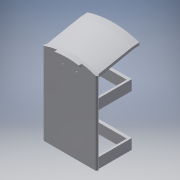
# Autodesk Inventor part: baseBateria
Saved by Autodesk Inventor 2017 (Build 210142000, 142)
## iProperties
Part Number: baseBateria
Material: Genérico
Document SubType Name: Modeling
Designer: Roberto
Density: 1 g/cm^3
Appearance: Valor por defecto
Author: Roberto
Autodesk Inventor part; units mm, degrees
ref_plane "XZ Plane" through (0, 0, 0) normal (0, 1, 0) x (-1, 0, 0)
ref_plane "XY Plane" through (0, 0, 0) normal (0, 0, 1) x (1, 0, 0)
sketch "Boceto1" plane through (0, 0, 0) normal (0, 1, 0) x (-1, 0, 0)
  line L0 (4.95, 0) -> (4.95, 8.1056)
  line L1 (-0.15, 0) -> (-0.15, 8.1056)
  arc A0 (4.95, 8.0532) -> (-0.15, 8.0532) centre (2.4, 1) ccw
  line L2 (-0.15, 0) -> (4.8, 0)
  line L3 (4.95, 0) -> (4.5, 0)
  line L4 (4.65, 0) -> (4.65, 1)
  line L5 (4.65, 1) -> (4.95, 1)
  line L6 (4.95, 5) -> (4.65, 5)
  line L7 (4.65, 5) -> (4.65, 6)
  line L8 (4.65, 6) -> (4.95, 6)
  line L9 (0.15, 0) -> (0.15, 1)
  line L10 (0.15, 1) -> (-0.15, 1)
  line L11 (-0.15, 5) -> (0.15, 5)
  line L12 (0.15, 5) -> (0.15, 6)
  line L13 (0.15, 6) -> (-0.15, 6)
  line L14 (0, 0) -> (1.4, 0)
  circle A1 centre (3.075, 7.5) radius 0.15
  circle A2 centre (1.725, 7.5) radius 0.15
  line L15 (2.55, 8.1985) -> (2.55, 0)
  line L16 (2.25, 8.1985) -> (2.25, 0)
  line L17 (0.9, 8.0485) -> (0.9, 0)
  line L18 (1.2, 8.1034) -> (1.2, 0)
  line L19 (3.9, 8.0485) -> (3.9, 0)
  line L20 (3.6, 8.1034) -> (3.6, 0)
  arc A3 (4.95, 7.7532) -> (-0.15, 7.7532) centre (2.4, 0.7) ccw
  line L21 (4.8, 0) -> (4.95, 0)
  line L22 (4.95, 8.0532) -> (4.95, 0)
  line L23 (4.95, 0) -> (-0.15, 0)
  constraints: 46 end point, 12 point on line, 10 point on circle, 4 centre point, 1 horizontal, 1 perpendicular, 1 vertical, 10 other
extrude "Extrusión1" add sketch "Boceto1" along normal blind 0.3
sketch "Boceto2" plane through (0, 0.3, 0) normal (0, 1, 0) x (1, 0, 0)
  line L0 (-4.8, 0) -> (-4.8, -8.1056)
  line L1 (0, 0) -> (0, -8.1056)
  arc A0 (-4.8, -8.1056) -> (0, -8.1056) centre (-2.4, -1) ccw
  line L2 (0, 0) -> (-4.8, 0)
  line L3 (-4.8, 0) -> (-4.5, 0)
  line L4 (-4.5, 0) -> (-4.5, -1)
  line L5 (-4.5, -1) -> (-4.8, -1)
  line L6 (-4.8, -5) -> (-4.5, -5)
  line L7 (-4.5, -5) -> (-4.5, -6)
  line L8 (-4.5, -6) -> (-4.8, -6)
  line L9 (-0.3, 0) -> (-0.3, -1)
  line L10 (-0.3, -1) -> (0, -1)
  line L11 (0, -5) -> (-0.3, -5)
  line L12 (-0.3, -5) -> (-0.3, -6)
  line L13 (-0.3, -6) -> (0, -6)
  line L14 (0, 0) -> (-1.4, 0)
  circle A1 centre (-3.075, -7.5) radius 0.15
  circle A2 centre (-1.725, -7.5) radius 0.15
  line L15 (-2.55, -7.8056) -> (-2.55, 0)
  line L16 (-2.25, -7.8056) -> (-2.25, 0)
  line L17 (-0.9, -7.8056) -> (-0.9, 0)
  line L18 (-1.2, -7.8056) -> (-1.2, 0)
  line L19 (-3.9, -7.8056) -> (-3.9, 0)
  line L20 (-3.6, -7.8056) -> (-3.6, 0)
  arc A3 (-4.8, -7.8056) -> (0, -7.8056) centre (-2.4, -0.7) ccw
  line L21 (-3.6, -7.8056) -> (-3.9, -7.8056)
  line L22 (-0.9, -7.8056) -> (-1.2, -7.8056)
  line L23 (-2.25, -7.8056) -> (-2.55, -7.8056)
  point P0 (0, 0)
  point P1 (-2.55, -8.1985)
  point P2 (-2.25, -8.1985)
  point P3 (-0.9, -8.0485)
  point P4 (-1.2, -8.1034)
  point P5 (-3.9, -8.0485)
  point P6 (-3.6, -8.1034)
  constraints: 46 end point, 11 point on line, 10 point on circle, 4 centre point, 3 horizontal, 12 other
extrude "Extrusión2" add sketch "Boceto2" along normal blind 0.3 contours L2 L20 L21 L19 | L2 L16 L23 L15 | L2 L17 L22 L18
sketch "Boceto7" plane through (0.15, 0, 0) normal (0, 0, -1) x (-1, 0, 0)
  line L0 (0.15, 0) -> (5.1, 0) projected
  line L1 (4.05, 0.3) -> (2.4, 0.3) projected
  line L2 (4.925, 0.15) -> (4.8, 0.3)
  line L3 (4.925, 0.15) -> (4.8, 0)
  line L4 (4.95, 0.3) -> (4.95, 3.55) projected
  line L5 (4.8, 0.3) -> (0, 0.3)
  line L6 (0.025, 0.15) -> (0, 0.3)
  line L7 (0.025, 0.15) -> (0.15, 0)
  line L8 (5.1, 0) -> (0.15, 0) projected
  line L9 (0.15, 0) -> (4.8, 0)
  point P0 (4.65, 0.3)
  constraints: 12 end point, 1 collinear, 1 horizontal, 1 other
extrude "Extrusión5" add sketch "Boceto7" against normal blind 9.2
sketch "Boceto8" plane through (0, 0.3, 0) normal (0, 1, 0) x (1, 0, 0)
  line L0 (-4.8, 0) -> (-4.8, -8.1056)
  line L1 (0, 0) -> (0, -8.1056)
  arc A0 (-4.8, -8.1056) -> (0, -8.1056) centre (-2.4, -1) ccw
  line L2 (0, 0) -> (-4.8, 0)
  line L3 (-4.8, 0) -> (-4.5, 0)
  line L4 (-4.5, 0) -> (-4.5, -1)
  line L5 (-4.5, -1) -> (-4.8, -1)
  line L6 (-4.8, -5) -> (-4.5, -5)
  line L7 (-4.5, -5) -> (-4.5, -6)
  line L8 (-4.5, -6) -> (-4.8, -6)
  line L9 (-0.3, 0) -> (-0.3, -1)
  line L10 (-0.3, -1) -> (0, -1)
  line L11 (0, -5) -> (-0.3, -5)
  line L12 (-0.3, -5) -> (-0.3, -6)
  line L13 (-0.3, -6) -> (0, -6)
  line L14 (0, 0) -> (-1.4, 0)
  circle A1 centre (-3.075, -7.5) radius 0.15
  circle A2 centre (-1.725, -7.5) radius 0.15
  line L15 (-2.55, -8.1985) -> (-2.55, 0)
  line L16 (-2.25, -8.1985) -> (-2.25, 0)
  line L17 (-0.9, -8.0485) -> (-0.9, 0)
  line L18 (-1.2, -8.1034) -> (-1.2, 0)
  line L19 (-3.9, -8.0485) -> (-3.9, 0)
  line L20 (-3.6, -8.1034) -> (-3.6, 0)
  arc A3 (-4.8, -7.8056) -> (0, -7.8056) centre (-2.4, -0.7) ccw
  arc A4 (-4.8, -8.1056) -> (0, -8.1056) centre (-2.4, -1) ccw
  arc A5 (-5.9319, -7.6163) -> (1.0681, -7.65) centre (-2.4, -1) ccw
  line L21 (1.0681, -7.65) -> (1.0681, -11.4465)
  line L22 (1.0681, -11.4465) -> (-5.9319, -11.4465)
  line L23 (-5.9319, -11.4465) -> (-5.9319, -7.6163)
  point P0 (0, 0)
  point P1 (0, 0)
  dimension "d20" = 7
  constraints: 46 end point, 14 point on circle, 11 point on line, 6 centre point, 2 perpendicular, 1 coincident, 1 vertical, 12 other
  measures "d20" distance of L21.end L22.end
extrude "Extrusión6" cut sketch "Boceto8" against normal blind 9.2 contours A0 A5 L21 L22 L23
sketch "Boceto12" plane through (0, 0, 0) normal (0, -1, 0) x (1, 0, 0)
  line L0 (0, 0) -> (0, 8.1056)
  line L1 (-4.8, 0) -> (-4.8, 8.1056)
  arc A0 (0, 8.1056) -> (-4.8, 8.1056) centre (-2.4, 1) ccw
  line L2 (-4.8, 0) -> (0, 0)
  line L3 (0, 0) -> (-0.3, 0)
  line L4 (-0.3, 0) -> (-0.3, 1)
  line L5 (-0.3, 1) -> (0, 1)
  line L6 (0, 5) -> (-0.3, 5)
  line L7 (-0.3, 5) -> (-0.3, 6)
  line L8 (-0.3, 6) -> (0, 6)
  line L9 (-4.5, 0) -> (-4.5, 1)
  line L10 (-4.5, 1) -> (-4.8, 1)
  line L11 (-4.8, 5) -> (-4.5, 5)
  line L12 (-4.5, 5) -> (-4.5, 6)
  line L13 (-4.5, 6) -> (-4.8, 6)
  line L14 (-4.8, 0) -> (-3.4, 0)
  circle A1 centre (-1.725, 7.5) radius 0.15
  circle A2 centre (-3.075, 7.5) radius 0.15
  line L15 (-2.25, 8.1985) -> (-2.25, 0)
  line L16 (-2.55, 8.1985) -> (-2.55, 0)
  line L17 (-3.9, 8.0485) -> (-3.9, 0)
  line L18 (-3.6, 8.1034) -> (-3.6, 0)
  line L19 (-0.9, 8.0485) -> (-0.9, 0)
  line L20 (-1.2, 8.1034) -> (-1.2, 0)
  arc A3 (0, 7.8056) -> (-4.8, 7.8056) centre (-2.4, 0.7) ccw
  point P0 (-4.8, 0)
  constraints: 40 end point, 11 point on line, 10 point on circle, 4 centre point, 12 other
extrude "Extrusión8" cut sketch "Boceto12" against normal blind 10 contours A1 | A2
sketch "Boceto14" plane through (0, 0, 0) normal (0, -1, 0) x (1, 0, 0)
  arc A0 (0.15, 8.0532) -> (-4.95, 8.0532) centre (-2.4, 1) ccw projected
  arc A1 (-1.2, 8.15) -> (-3.6, 8.15) centre (-2.4, 1) ccw
  line L0 (-1.2, 8.4034) -> (-1.2, 8.15)
  line L1 (-3.6, 8.4034) -> (-3.6, 8.15)
  arc A2 (-1.2, 8.4034) -> (-3.6, 8.4034) centre (-2.4, 1) ccw
  point P0 (0, 0)
  point P1 (0, 8.1056)
  point P2 (-4.8, 8.1056)
  dimension "d34" = 0.25
  constraints: 6 point on circle, 4 end point, 2 centre point, 1 concentric
  measures "d34" radial gap between concentric circles of A0 A1
extrude "Extrusión10" add sketch "Boceto14" along normal blind 0.3
chamfer "Chaflán1" distance 0.2 angle 45 1 edges at (-2.4, -0.3, 8.25)
sketch "Boceto17" plane through (0, 0.3, 0) normal (0, 1, 0) x (1, 0, 0)
  line L0 (-2.25, 0) -> (-2.55, 0) projected
  line L1 (0.15, 0) -> (-4.95, 0) projected
  line L2 (0.15, 0) -> (-0.05, 0)
  line L3 (-4.75, 0) -> (-4.95, 0)
  line L4 (0.15, 0) -> (0.15, -1)
  line L5 (0.15, -8.0532) -> (0.15, 0) projected
  line L6 (0.15, -1) -> (-0.05, -1)
  line L7 (-0.05, -1) -> (-0.05, 0)
  line L8 (-0.05, 0) -> (0.15, 0)
  line L9 (0.15, 0) -> (0.15, -1)
  line L10 (-4.95, 0) -> (-4.95, -1)
  line L11 (-4.95, -1) -> (-4.75, -1)
  line L12 (-4.75, -1) -> (-4.75, 0)
  line L13 (-4.75, 0) -> (-4.95, 0)
  line L14 (-4.95, 0) -> (-4.95, -1)
  line L15 (-4.95, 0) -> (-4.95, -5)
  line L16 (-4.95, 0) -> (-4.95, -8.0532) projected
  line L17 (-4.95, -5) -> (-4.75, -5)
  line L18 (-4.75, -5) -> (-4.75, -6)
  line L19 (-4.75, -6) -> (-4.95, -6)
  line L20 (-4.95, -6) -> (-4.95, -5)
  line L21 (0.15, 0) -> (0.15, -5)
  line L22 (0.15, -5) -> (0.15, -6)
  line L23 (0.15, -6) -> (-0.05, -6)
  line L24 (-0.05, -6) -> (-0.05, -5)
  line L25 (-0.05, -5) -> (0.15, -5)
  point P0 (0, 0)
  dimension "d55" = 1
  dimension "d56" = 1
  dimension "d57" = 5
  dimension "d58" = 0.2
  dimension "d59" = 1
  dimension "d60" = 0.2
  dimension "d61" = 5
  dimension "d62" = 1
  dimension "d63" = 0.2
  dimension "d64" = 1
  constraints: 44 end point, 9 point on line, 5 parallel, 3 horizontal, 3 perpendicular, 1 collinear, 1 vertical
  measures "d55" distance of L1.start L4.end
  measures "d56" distance of L1.end L10.end
  measures "d57" distance of L13.end L15.end
  measures "d58" distance of L15.end L17.end
  measures "d59" distance of L17.end L18.end
  measures "d60" distance of L18.end L19.end
  measures "d61" distance of L8.end L21.end
  measures "d62" distance of L21.end L22.end
  measures "d63" distance of L22.end L23.end
  measures "d64" distance of L23.end L24.end
extrude "Extrusión12" add sketch "Boceto17" along normal blind 3.25
sketch "Boceto18" plane through (0.15, 0.3, 5) normal (0, 0, -1) x (-1, 0, 0)
  line L0 (0, 0) -> (0.2, 0) projected
  line L1 (0, 0) -> (0, 3.25) projected
  line L2 (0.2, 3.25) -> (0, 3.25) projected
  line L3 (0.2, 0) -> (0.2, 3.25) projected
  line L4 (4.9, 0) -> (5.1, 0) projected
  line L5 (4.9, 0) -> (4.9, 3.25) projected
  line L6 (5.1, 3.25) -> (4.9, 3.25) projected
  line L7 (5.1, 0) -> (5.1, 3.25) projected
  line L8 (0.2, 3.25) -> (0.2, 2.95)
  line L9 (0.2, 0) -> (0.2, 3.25) projected
  line L10 (4.9, 0) -> (4.9, 3.25) projected
  line L11 (4.9, 3.25) -> (0.2, 3.25)
  line L12 (0.2, 3.25) -> (0.2, 2.95)
  line L13 (0.2, 2.95) -> (4.9, 2.95)
  line L14 (4.9, 2.95) -> (4.9, 3.25)
  point P0 (0.15, -0.3)
  dimension "d67" = 0.3
  constraints: 10 end point, 2 parallel, 1 horizontal, 1 perpendicular, 1 point on line
  measures "d67" distance of L2.start L8.end
extrude "Extrusión13" add sketch "Boceto18" against normal blind 1 contours L3 L11 L5 L13
sketch "Boceto19" plane through (0.15, 0, 0) normal (0, 0, -1) x (-1, 0, 0)
  line L0 (5.1, 0.3) -> (4.9, 0.3) projected
  line L1 (5.1, 0.3) -> (5.1, 3.55) projected
  line L2 (0, 3.55) -> (5.1, 3.55) projected
  line L3 (0, 0.3) -> (0, 3.55) projected
  line L4 (0.2, 0.3) -> (0, 0.3) projected
  line L5 (0.2, 0.3) -> (0.2, 3.25) projected
  line L6 (0.2, 3.25) -> (4.9, 3.25) projected
  line L7 (4.9, 0.3) -> (4.9, 3.25) projected
  line L8 (5.1, 3.55) -> (4.9, 3.55) projected
  line L9 (0.2, 3.25) -> (4.9, 3.25)
  line L10 (4.9, 3.25) -> (4.9, 3.55)
  line L11 (4.9, 3.55) -> (0.2, 3.55)
  line L12 (0.2, 3.55) -> (0.2, 3.25)
  point P0 (0.15, 0)
  constraints: 8 end point, 2 parallel, 1 horizontal, 1 perpendicular
extrude "Extrusión14" add sketch "Boceto19" against normal blind 1 contours L6 L12 L2 L10
ref_plane "Plano de trabajo2" through (-2.4, 0, 0) normal (1, 0, 0) x (0, 1, 0)
sketch "Boceto20" plane through (-2.4, 0, 0) normal (1, 0, 0) x (0, 1, 0)
  line L0 (0.6, 8.1985) -> (0.6, 0) projected
  line L1 (3.5908, 9.1113) -> (3.6479, 8.874)
  line L2 (0.3, 8.2233) -> (3.6479, 8.874)
  line L3 (3.6479, 8.874) -> (0.3, 8.2233)
  line L4 (3.5908, 9.1113) -> (0.3, 8.5)
  line L5 (3.5908, 9.1113) -> (0.3, 8.5)
  line L6 (0, 0) -> (0.3056, 0)
  line L7 (0.2767, 0) -> (0, 0)
  line L8 (0, 0) -> (0.3056, 0)
  line L9 (0.3, 8.5) -> (0.3, -6.5)
  arc A0 (12.685, 1) -> (11.6118, 4.6054) centre (3.0813, 0.1036) ccw
  line L10 (12.9279, 1) -> (12.685, 1)
  arc A1 (12.9279, 1) -> (11.8616, 4.6496) centre (3.0813, 0.1036) ccw
  arc A2 (4.3, 9.1546) -> (3.5908, 9.1113) centre (4.4538, 0.8142) ccw
  line L11 (0.3, 8.0532) -> (0.3, 8.5) projected
  line L12 (4.3, 8.9127) -> (4.3, 9.1546)
  arc A3 (11.647, 4.5382) -> (11.6118, 4.6054) centre (4.4538, 0.8142) ccw
  arc A4 (4.3, 8.9127) -> (3.6479, 8.874) centre (4.4538, 0.8142) ccw
  line L13 (0.3, 8.5) -> (0.3, 8.2233)
  line L14 (0.3, 8.2233) -> (3.6479, 8.874)
  arc A5 (4.3, 8.9127) -> (3.6479, 8.874) centre (4.4537, 0.8144) ccw
  arc A6 (4.3, 9.1546) -> (3.5908, 9.1113) centre (4.4538, 0.8142) ccw
  line L15 (3.5908, 9.1113) -> (0.3, 8.5)
  dimension "d73" = 15
  constraints: 28 end point, 15 point on circle, 7 centre point, 4 collinear, 2 coincident, 2 horizontal, 1 concentric, 1 vertical
  measures "d73" distance of L9.start L9.end
revolve "Revolución4" add sketch "Boceto20" angle 43 mid plane about axis through (-2.4, 12.9279, 1) along (0, -1, 0)
sketch "Boceto21" plane through (0.15, 0.3, 7.7582) normal (0, -1, 0) x (1, 0, 0)
  line L0 (0, 0.295) -> (0, 0) projected
  line L1 (-5.1, 0) -> (-5.1, 0.295) projected
  line L2 (-5.1, 0) -> (-5.1, -0.5126)
  line L3 (-5.1, -0.5126) -> (-6.7261, -0.5126)
  line L4 (-6.7261, -0.5126) -> (-6.7261, 2.8474)
  line L5 (-6.7261, 2.8474) -> (-5.1, 2.8474)
  line L6 (-5.1, 2.8474) -> (-5.1, 0)
  line L7 (0, 0) -> (0, 2.8474)
  line L8 (0, 2.8474) -> (2.3342, 2.8474)
  line L9 (2.3342, 2.8474) -> (2.3342, -0.5126)
  line L10 (2.3342, -0.5126) -> (0, -0.5126)
  line L11 (0, 0) -> (0, -0.5126)
  point P0 (-0.15, -7.7582)
  constraints: 20 end point, 6 perpendicular, 6 point on line, 1 parallel, 1 vertical
extrude "Extrusión15" cut sketch "Boceto21" against normal blind 10000
sketch "Boceto23" plane through (0.15, 0, 0) normal (0, 0, -1) x (-1, 0, 0)
  line L0 (0, 0) -> (4.8, 0)
  line L1 (3.9, 0.3) -> (4.5, 0.3)
  line L2 (4.8, 0.3) -> (0, 0.3)
  line L3 (-0.125, 0.15) -> (0, 0.3)
  line L4 (-0.125, 0.15) -> (0, 0)
  line L5 (4.8, 0) -> (0, 0)
  line L6 (0, 0) -> (4.8, 0)
  line L7 (5.1, 0) -> (5.1, 3.55) projected
  line L8 (5.225, 0.15) -> (5.1, 0.3)
  line L9 (5.225, 0.15) -> (5.1, 0)
  line L10 (5.1, 0.3) -> (0, 0.3)
  line L11 (0, 0) -> (0, 3.55) projected
  line L12 (0, 0) -> (5.1, 0) projected
  line L13 (0, 0) -> (5.1, 0)
  line L14 (-0.125, 0.15) -> (0, 0.3)
  line L15 (0, 0.3) -> (5.1, 0.3)
  line L16 (5.1, 0) -> (5.1, 0.3) projected
  line L17 (5.1, 0.3) -> (5.225, 0.15)
  line L18 (5.225, 0.15) -> (5.1, 0)
  line L19 (5.1, 0) -> (0, 0)
  line L20 (0, 0) -> (-0.125, 0.15)
  point P0 (0.15, 0)
  constraints: 34 end point, 3 collinear, 3 perpendicular, 2 horizontal
extrude "Extrusión16" add sketch "Boceto23" against normal blind 10
sketch "Boceto24" plane through (-2.4, 0.3, 1) normal (0, 1, 0) x (1, 0, 0)
  arc A0 (-2.55, -7.0532) -> (2.55, -7.0532) centre (0, 0) ccw projected
  line L0 (0, -10.5) -> (3.5, -10.5)
  line L1 (3.5, -10.5) -> (3.5, -6.6332)
  line L2 (0, -10.5) -> (-3.5, -10.5)
  line L3 (-3.5, -10.5) -> (-3.5, -6.6332)
  arc A1 (-2.55, -7.0532) -> (2.55, -7.0532) centre (0, 0) ccw
  arc A2 (-3.5, -6.6332) -> (3.5, -6.6332) centre (0, 0) ccw
  point P0 (2.4, 1)
  dimension "d81" = 3.5
  dimension "d82" = 3.5
  constraints: 8 end point, 4 point on circle, 2 centre point, 2 perpendicular, 1 coincident, 1 horizontal
  measures "d81" distance of L0.start L0.end
  measures "d82" distance of L0.start L2.end
extrude "Extrusión17" cut sketch "Boceto24" against normal blind 10
sketch "Boceto25" plane through (0, 0.3, 0) normal (0, 1, 0) x (1, 0, 0)
  line L0 (-0.15, 0) -> (-5.1, 0)
  circle A0 centre (-3.075, -7.5) radius 0.15
  circle A1 centre (-1.725, -7.5) radius 0.15
  line L1 (-4.95, -8.0532) -> (-4.95, 0)
  line L2 (-4.95, 0) -> (-4.95, -1) projected
  circle A2 centre (-1.725, -7.5) radius 0.075
  circle A3 centre (-3.075, -7.5) radius 0.075
  point P0 (0, 0)
  point P1 (-1.7, 0)
  point P2 (-2.85, 0)
  point P3 (-2.55, 0)
  point P4 (-1.2, 0)
  point P5 (-1.5, 0)
  point P6 (-4.2, 0)
  point P7 (-3.9, 0)
  dimension "d88" = 0.15
  dimension "d89" = 0.15
  constraints: 4 centre point, 2 coincident, 2 end point, 10 other
  measures "d88" diameter of A2
  measures "d89" diameter of A3
extrude "Extrusión18" cut sketch "Boceto25" against normal blind 10 contours A2 | A3
